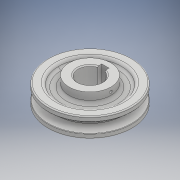
# Autodesk Inventor part: 2강V-벨트풀리
Saved by Autodesk Inventor 2018.3 (Build 223284000, 284)
## iProperties
Created: 2019-10-10
Part Number: 2강V-벨트풀리
Material: 일반
Document SubType Name: Modeling
Designer: MyTool
Density: 1 g/cm^3
Appearance: 기본값
Author: MyTool
Autodesk Inventor part; units mm, degrees
ref_plane "YZ Plane" through (0, 0, 0) normal (1, 0, 0) x (0, 1, 0)
ref_plane "XZ Plane" through (0, 0, 0) normal (0, 1, 0) x (-1, 0, 0)
ref_plane "XY Plane" through (0, 0, 0) normal (0, 0, 1) x (1, 0, 0)
sketch "스케치1" plane through (0, 0, 0) normal (1, 0, 0) x (0, 1, 0)
  line L0 (0, 0) -> (0, 9.5)
  line L1 (0, 9.5) -> (40.2, 9.5)
  line L2 (40.2, 9.5) -> (40.2, 4.8773)
  line L3 (40.2, 4.8773) -> (37.5, 4)
  line L4 (37.5, 4) -> (31.2, 1.953)
  line L5 (31.2, 1.953) -> (31.2, 0)
  line L6 (31.2, 0) -> (0, 0)
  dimension "d1" = 37.5
  dimension "d2" = 4
  dimension "d3" = 6.3
  dimension "d4" = 9.5
  dimension "d5" = 2.7
  dimension "d7" = 18
  constraints: 14 end point, 3 perpendicular, 1 parallel, 1 point on line, 1 vertical
  measures "d1" distance from line of L0 L3.end
  measures "d2" distance from line of L6 L3.end
  measures "d3" horizontal distance of L4.end L3.end
  measures "d4" distance between parallel lines of L6 L1
  measures "d5" distance from line of L3.end L2
  measures "d7" angle of L6 L4
revolve "회전1" add sketch "스케치1" angle 360 about axis through (0, 0, 0) along (0, 0, 1)
mirror "미러1" about plane through (0, 0, 0) normal (0, 0, -1) of "회전1"
fillet "모깎기1" radius 1 2 edges at (0, -40.2, 9.5) (0, -40.2, -9.5)
fillet "모깎기2" radius 0.5 2 edges at (0, -40.2, 4.8773) (0, -40.2, -4.8773)
fillet "모깎기3" radius 1 2 edges at (0, -31.2, 1.953) (0, -31.2, -1.953)
sketch "스케치2" plane through (0, 0, 9.5) normal (0, 0, 1) x (1, 0, 0)
  circle A0 centre (0, 0) radius 20
  dimension "d11" = 40
  constraints: 1 centre point, 1 coincident
  measures "d11" diameter of A0
extrude "돌출1" add sketch "스케치2" along normal blind 6
sketch "스케치3" plane through (0, 0, 15.5) normal (0, 0, 1) x (1, 0, 0)
  circle A0 centre (0, 0) radius 11.5
  line L0 (-3.5, 14.8) -> (-3.5, 0)
  line L1 (-3.5, 0) -> (3.5, 0)
  line L2 (3.5, 0) -> (3.5, 14.8)
  line L3 (3.5, 14.8) -> (-3.5, 14.8)
  line L4 (-3.5, 14.8) -> (3.5, 0) construction
  line L5 (-3.5, 0) -> (3.5, 14.8) construction
  point P0 (0, 7.4)
  dimension "d14" = 23
  dimension "d15" = 7
  dimension "d16" = 3.5
  dimension "d17" = 14.8
  dimension "d18" = 11.5
  constraints: 12 end point, 2 midpoint, 2 parallel, 1 centre point, 1 coincident, 1 perpendicular, 1 vertical
  measures "d14" diameter of A0
  measures "d15" distance of L2.end L0.start
  measures "d16" distance from line of A0.centre L0
  measures "d17" distance between parallel lines of L1 L3
  measures "d18" distance edge to line of A0 L1
extrude "돌출2" cut sketch "스케치3" against normal up to next
chamfer "모따기1" distance 1 angle 45 2 edges at (0, -11.5, 15.5) (0, -11.5, -9.5)
sketch "스케치4" plane through (0, 0, -9.5) normal (0, 0, -1) x (-1, 0, 0)
  circle A0 centre (0, 0) radius 30
  circle A1 centre (0, 0) radius 20
  dimension "d24" = 60
  dimension "d25" = 40
  constraints: 2 centre point, 2 coincident
  measures "d24" diameter of A0
  measures "d25" diameter of A1
extrude "돌출3" cut sketch "스케치4" against normal blind 4
mirror "미러2" about plane through (0, 0, 0) normal (0, 0, 1) of "돌출3"
fillet "모깎기4" radius 3 6 edges at (30, 0, 9.5) (30, 0, 5.5) (20, 0, 5.5) (20, 0, -5.5) (30, 0, -5.5) (30, 0, -9.5)
sketch "스케치5" plane through (0, 0, 0) normal (1, 0, 0) x (0, 1, 0)
  circle A0 centre (0, 11.5) radius 1.5
  line L0 (20, 15.5) -> (-20, 15.5) projected
  point P0 (0, 0)
  dimension "d29" = 3
  dimension "d30" = 4
  constraints: 1 centre point
  measures "d29" diameter of A0
  measures "d30" distance from line of A0.centre L0
hole "구멍1" at (0, 0, 11.5) direction (1, 0, 0) diameter 2.459 end through all thread size "M3x0.5" class "6H" standard "ANSI Metric M Profile"
